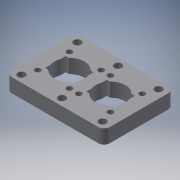
# Autodesk Inventor part: cylinder frame
Saved by Autodesk Inventor 2016 (Build 200138000, 138)
## iProperties
Created: 2017-06-14
Part Number: cylinder frame
Material: Generic
Document SubType Name: Modeling
Designer: RMcComber
Density: 1 g/cm^3
Appearance: Default
Author: RMcComber
Autodesk Inventor part; units mm, degrees
ref_plane "YZ Plane" through (0, 0, 0) normal (1, 0, 0) x (0, 1, 0)
ref_plane "XZ Plane" through (0, 0, 0) normal (0, 1, 0) x (-1, 0, 0)
ref_plane "XY Plane" through (0, 0, 0) normal (0, 0, 1) x (1, 0, 0)
sketch "Sketch1" plane through (0, 0, 0) normal (0, 0, 1) x (1, 0, 0)
  line L0 (-22, 0) -> (22, 0) construction
  circle A0 centre (-22, 0) radius 16
  circle A1 centre (22, 0) radius 16
  line L1 (43.5, -30) -> (-43.5, -30) construction
  line L2 (-43.5, -30) -> (-43.5, 30) construction
  line L3 (-43.5, 30) -> (43.5, 30) construction
  line L4 (43.5, 30) -> (43.5, -30) construction
  line L5 (43.5, -30) -> (-43.5, 30) construction
  line L6 (-43.5, -30) -> (43.5, 30) construction
  circle A2 centre (-43.5, 30) radius 4
  circle A3 centre (0, 30) radius 4
  circle A4 centre (43.5, 30) radius 4
  circle A5 centre (43.5, -30) radius 4
  circle A6 centre (-43.5, -30) radius 4
  circle A7 centre (0, -30) radius 4
  line L7 (-52.5, -37.5) -> (52.5, -37.5)
  line L8 (52.5, -37.5) -> (52.5, 37.5)
  line L9 (52.5, 37.5) -> (-52.5, 37.5)
  line L10 (-52.5, 37.5) -> (-52.5, -37.5)
  line L11 (-52.5, -37.5) -> (52.5, 37.5) construction
  line L12 (52.5, -37.5) -> (-52.5, 37.5) construction
  line L13 (-5, -17) -> (-39, -17) construction
  line L14 (-39, -17) -> (-39, 17) construction
  line L15 (-39, 17) -> (-5, 17) construction
  line L16 (-5, 17) -> (-5, -17) construction
  line L17 (-5, -17) -> (-39, 17) construction
  line L18 (-39, -17) -> (-5, 17) construction
  line L19 (39, -17) -> (5, -17) construction
  line L20 (5, -17) -> (5, 17) construction
  line L21 (5, 17) -> (39, 17) construction
  line L22 (39, 17) -> (39, -17) construction
  line L23 (39, -17) -> (5, 17) construction
  line L24 (5, -17) -> (39, 17) construction
  circle A8 centre (-39, 17) radius 3
  circle A9 centre (-39, -17) radius 3
  circle A10 centre (-5, -17) radius 3
  circle A11 centre (-5, 17) radius 3
  circle A12 centre (5, 17) radius 3
  circle A13 centre (5, -17) radius 3
  circle A14 centre (39, -17) radius 3
  circle A15 centre (39, 17) radius 3
  point P0 (0, 0)
  point P1 (0, 0)
  dimension "d0" = 60
  dimension "d1" = 87
  dimension "d2" = 44
  dimension "d3" = 32
  dimension "d4" = 8
  dimension "d5" = 105
  dimension "d6" = 75
  dimension "d10" = 34
  dimension "d11" = 6
  constraints: 50 end point, 16 centre point, 15 coincident, 13 equal radius, 11 midpoint, 8 parallel, 7 perpendicular, 5 horizontal
  measures "d0" distance of L1.end L2.end
  measures "d1" distance of L2.end L3.end
  measures "d2" distance of L0.start L0.end
  measures "d3" diameter of A0
  measures "d4" diameter of A2
  measures "d5" distance of L8.end L9.end
  measures "d6" distance of L7.end L8.end
  measures "d10" distance of L13.end L14.end
  measures "d11" diameter of A8
extrude "Extrusion1" add sketch "Sketch1" along normal blind 15
fillet "Fillet1" radius 6 4 edges at (-52.5, 37.5, 7.5) (52.5, 37.5, 7.5) (52.5, -37.5, 7.5) (-52.5, -37.5, 7.5)
sketch "Sketch2" plane through (0, 0, 15) normal (0, 0, 1) x (1, 0, 0)
  circle A0 centre (22, 0) radius 16 projected
  circle A1 centre (-22, 0) radius 16 projected
  line L0 (37, -11) -> (7, -11)
  line L1 (7, -11) -> (7, 11)
  line L2 (7, 11) -> (37, 11)
  line L3 (37, 11) -> (37, -11)
  line L4 (37, -11) -> (7, 11) construction
  line L5 (7, -11) -> (37, 11) construction
  line L6 (-37, -11) -> (-7, -11)
  line L7 (-7, -11) -> (-7, 11)
  line L8 (-7, 11) -> (-37, 11)
  line L9 (-37, 11) -> (-37, -11)
  line L10 (-37, -11) -> (-7, 11) construction
  line L11 (-7, -11) -> (-37, 11) construction
  point P0 (0, 0)
  dimension "d12" = 22
  dimension "d13" = 30
  constraints: 24 end point, 4 midpoint, 4 parallel, 2 equal length, 2 horizontal, 2 perpendicular
  measures "d12" distance of L6.end L7.end
  measures "d13" distance of L7.end L8.end
extrude "Extrusion2" cut sketch "Sketch2" against normal through all contours L3 A0 L0 L1 L2 | A0 L2 L3 | L3 L0 A0 | A0 L1 L2 | L0 L1 A0 | L7 A1 L6 L9 L8 | A1 L8 L7 | L7 L6 A1 | A1 L9 L8 | L6 L9 A1
sketch "Sketch3" plane through (0, 0, 15) normal (0, 0, 1) x (1, 0, 0)
  arc A0 (-10.381, 11) -> (-33.619, 11) centre (-22, 0) ccw construction
  arc A1 (33.619, 11) -> (10.381, 11) centre (22, 0) ccw construction
  line L0 (-22, -30) -> (22, -30) construction
  line L1 (22, -30) -> (22, 30) construction
  line L2 (22, 30) -> (-22, 30) construction
  line L3 (-22, 30) -> (-22, -30) construction
  line L4 (-22, -30) -> (22, 30) construction
  line L5 (22, -30) -> (-22, 30) construction
  circle A2 centre (0, 30) radius 4 construction
  circle A3 centre (-22, 30) radius 4
  circle A4 centre (22, 30) radius 4
  circle A5 centre (22, -30) radius 4
  circle A6 centre (-22, -30) radius 4
  point P0 (0, 0)
  dimension "d16" = 8
  constraints: 12 end point, 5 coincident, 4 centre point, 4 midpoint, 3 equal radius, 2 parallel, 1 horizontal, 1 perpendicular
  measures "d16" diameter of A6
extrude "Extrusion3" cut sketch "Sketch3" against normal through all
body "Solid1"
